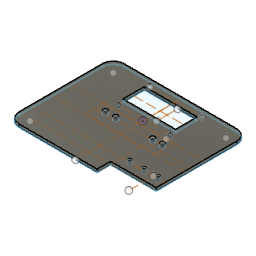
Frente carcasa (Autodesk Fusion 360 design; units mm, degrees)
Autodesk Fusion 360 part; units mm, degrees
sketch "Sketch1" plane through (0, 0, 0) normal (0, 0, 1) x (1, 0, 0)
  line L0 (-105, 70) -> (105, 70)
  line L1 (125, 50) -> (125, -100)
  line L2 (-125, -105) -> (-125, 50)
  line L3 (0, 0) -> (0, -125) construction
  line L4 (0, 70) -> (0, 0) construction
  line L5 (125, -100) -> (-125, -100) construction
  line L6 (99.0375, -125) -> (99.0375, -79) construction
  line L7 (125, -79) -> (-125, -79) construction
  circle A0 centre (108, -79) radius 2.5
  line L8 (108, -79) -> (82, -79) construction
  circle A1 centre (82, -79) radius 2.5
  line L9 (82, -79) -> (55, -79) construction
  circle A2 centre (55, -79) radius 2.5
  line L10 (125, -100) -> (40, -100)
  line L11 (40, -100) -> (40, -125)
  line L12 (40, -125) -> (40, -32) construction
  line L13 (40, -32) -> (125, -32) construction
  line L14 (125, -42.4326) -> (-125, -42.4326) construction
  line L15 (0, -7.4326) -> (65, -7.4326) construction
  line L16 (65, -7.4326) -> (65, -42.4326) construction
  line L17 (65, -42.4326) -> (-65, -42.4326) construction
  line L18 (-65, -42.4326) -> (-65, -7.4326) construction
  line L19 (-65, -7.4326) -> (0, -7.4326) construction
  line L20 (65, -22.4326) -> (-65, -22.4326) construction
  circle A3 centre (59, -22.4326) radius 4
  circle A4 centre (41, -22.4326) radius 4
  line L21 (50.7951, -22.4326) -> (50.7951, -7.4326) construction
  line L22 (-65, -26.2761) -> (-47, -26.2761) construction
  line L23 (-47, -26.2761) -> (-47, -22.4326) construction
  circle A5 centre (-47, -22.4326) radius 4
  line L24 (-47, -26.2761) -> (-28, -26.2761) construction
  line L25 (-28, -26.2761) -> (-28, -22.4326) construction
  circle A6 centre (-28, -22.4326) radius 4
  line L26 (-49, 62.2518) -> (49, 62.2518) construction
  line L27 (49, 2.2518) -> (-49, 2.2518) construction
  line L28 (-49, 32.2518) -> (49, 32.2518) construction
  line L29 (0, 62.2518) -> (0, 2.2518) construction
  line L30 (12.9393, 32.2518) -> (12.9393, 52.2518) construction
  line L31 (12.9393, 32.2518) -> (12.9393, 12.2518) construction
  line L32 (49, 52.2518) -> (-49, 52.2518)
  line L33 (49, 12.2518) -> (-49, 12.2518)
  circle A7 centre (-48, 61.2518) radius 0.75
  line L34 (49, 61.2518) -> (48, 61.2518) construction
  line L35 (48, 62.2518) -> (48, 61.2518) construction
  circle A8 centre (48, 61.2518) radius 0.75
  line L36 (49, 3.2518) -> (48, 3.2518) construction
  line L37 (48, 3.2518) -> (48, 2.2518) construction
  circle A9 centre (48, 3.2518) radius 0.75
  line L38 (-48, 2.2518) -> (-48, 3.2518) construction
  line L39 (-49, 3.2518) -> (-48, 3.2518) construction
  circle A10 centre (-48, 3.2518) radius 0.75
  arc A11 (-105, 70) -> (-125, 50) centre (-105, 50) ccw
  arc A12 (125, 50) -> (105, 70) centre (105, 50) ccw
  arc A13 (-125, -105) -> (-105, -125) centre (-105, -105) ccw
  line L40 (-125, -7.4326) -> (125, -7.4326) construction
  line L41 (49, 62.2518) -> (49, 61.2518)
  line L42 (49, 52.2518) -> (49, 62.2518) construction
  line L43 (-49, 52.2518) -> (-49, 62.2518) construction
  line L44 (-49, 2.2518) -> (-49, 3.2518)
  line L45 (-49, 12.2518) -> (-49, 52.2518)
  line L46 (-49, 12.2518) -> (-49, 3.2518) construction
  line L47 (49, 52.2518) -> (49, 12.2518)
  line L48 (49, 3.2518) -> (49, 2.2518)
  line L49 (49, 12.2518) -> (49, 2.2518) construction
  line L50 (40, -125) -> (-105, -125)
  dimension "d12" = 46
  dimension "d13" = 17
  dimension "d14" = 5
  dimension "d16" = 5
  dimension "d18" = 5
  dimension "d19" = 85
  dimension "d20" = 93
  dimension "d21" = 65
  dimension "d22" = 130
  dimension "d33" = 8
  dimension "d34" = 8
  dimension "d37" = 15
  dimension "d38" = 18
  dimension "d39" = 8
  dimension "d40" = 19
  dimension "d41" = 8
  dimension "d42" = 98
  dimension "d43" = 60
  dimension "d44" = 20
  dimension "d45" = 20
  dimension "d46" = 98
  dimension "d47" = 98
  dimension "d50" = 1.5
  dimension "d52" = 1
  dimension "d53" = 1
  dimension "d54" = 1.5
  dimension "d56" = 1
  dimension "d57" = 1.5
  dimension "d59" = 1
  dimension "d60" = 1.5
  dimension "d67" = 20
  dimension "d68" = 20
  dimension "d69" = 20
  constraint horizontal L0
  constraint vertical L1
  constraint vertical L2
  constraint coincident L3.start L4.end
  constraint coincident L2 L5.end
  constraint perpendicular L2 L5
  constraint coincident L1 L7.start
  constraint coincident L2 L7.end
  constraint perpendicular L2 L7
  constraint coincident A0.centre L8.start
  constraint parallel L7 L8
  constraint coincident L8.end A1.centre
  constraint parallel L7 L9
  constraint coincident L9.end A2.centre
  constraint perpendicular L1 L10
  constraint perpendicular L5 L12
  constraint coincident L1 L13.end
  constraint perpendicular L1 L13
  constraint coincident L1 L14.start
  constraint coincident L2 L14.end
  constraint perpendicular L2 L14
  constraint perpendicular L3 L15
  constraint coincident L14 L16.end
  constraint perpendicular L14 L16
  constraint perpendicular L3 L17
  constraint perpendicular L3 L19
  constraint coincident L16 L20.start
  constraint coincident L18 L20.end
  constraint perpendicular L18 L20
  constraint coincident L20 A3.centre
  constraint coincident L20 A4.centre
  constraint coincident L20 L21.start
  constraint perpendicular L20 L21
  constraint coincident L18 L22.start
  constraint perpendicular L18 L22
  constraint coincident L20 L23.end
  constraint perpendicular L20 L23
  constraint coincident L23.end A5.centre
  constraint perpendicular L23 L24
  constraint coincident L20 L25.end
  constraint perpendicular L20 L25
  constraint coincident L25.end A6.centre
  constraint horizontal L26
  constraint vertical L41
  constraint horizontal L27
  constraint vertical L44
  constraint midpoint L26 L29.start
  constraint midpoint L27 L29.end
  constraint coincident L28 L30.start
  constraint perpendicular L28 L30
  constraint vertical L31
  constraint coincident L32.start L41
  constraint perpendicular L32 L41
  constraint coincident L33.start L41
  constraint perpendicular L33 L41
  constraint perpendicular L34 L41
  constraint coincident L26 L35.start
  constraint perpendicular L26 L35
  constraint coincident L34.end L35.end
  constraint coincident L36.start L41
  constraint perpendicular L36 L41
  constraint coincident L27 L37.end
  constraint perpendicular L27 L37
  constraint coincident L36.end L37.start
  constraint coincident L27 L38.start
  constraint perpendicular L27 L38
  constraint perpendicular L38 L39
  constraint coincident L38.end L39.end
  constraint coincident L0 L4.start
  constraint tangent L0 A11
  constraint tangent L2 A11
  constraint tangent L0 A12
  constraint tangent L1 A12
  constraint tangent L2 A13
  constraint coincident L2 L40.start
  constraint coincident L1 L40.end
  constraint perpendicular L1 L40
  constraint collinear L41 L47
  constraint coincident L28.end L41
  constraint coincident L28.start L44
  constraint perpendicular L26 L43
  constraint collinear L44 L45
  constraint collinear L47 L48
  measures "d12" distance of L6.start L6.end
  measures "d13" distance of L7.start A0.centre
  measures "d14" diameter of A0
  measures "d16" diameter of A1
  measures "d18" diameter of A2
  measures "d19" distance of L1.end L10.end
  measures "d20" distance of L11.end L12.end
  measures "d21" distance of L15.start L15.end
  measures "d22" distance of L16.end L17.end
  measures "d33" diameter of A3
  measures "d34" diameter of A4
  measures "d37" distance of L21.start L21.end
  measures "d38" distance of L22.start L22.end
  measures "d39" diameter of A5
  measures "d40" distance of L22.end L24.end
  measures "d41" diameter of A6
  measures "d42" distance of L26.start L26.end
  measures "d43" distance of L26.start L27.end
  measures "d44" distance of L30.start L30.end
  measures "d45" distance of L30.start L31.end
  measures "d46" distance of L32.start L32.end
  measures "d47" distance of L33.start L33.end
  measures "d50" diameter of A7
  measures "d52" distance of L34.start L34.end
  measures "d53" distance of L35.start L34.end
  measures "d54" diameter of A8
  measures "d56" distance of L36.start L36.end
  measures "d57" diameter of A9
  measures "d59" distance of L38.start L38.end
  measures "d60" diameter of A10
  measures "d67" radius of A11
  measures "d68" radius of A12
  measures "d69" radius of A13
extrude "Extruir1" add sketch "Sketch1" along normal blind 5
